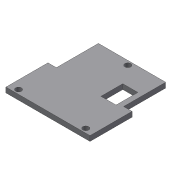
# Autodesk Inventor part: arm_0_bottom_case
Saved by Autodesk Inventor 2018 (Build 220112000, 112)
## iProperties
Created: 2017-12-04
Part Number: arm_0_bottom_case
Material: Generic
Document SubType Name: Modeling
Designer: Bardo91
Density: 1 g/cm^3
Appearance: Default
Mass: 6.66341 g
Surface Area: 51.4123 cm^2
Volume: 6.66341 cm^3
Author: Bardo91
Autodesk Inventor part; units mm, degrees
ref_plane "YZ Plane" through (0, 0, 0) normal (1, 0, 0) x (0, 1, 0)
ref_plane "XZ Plane" through (0, 0, 0) normal (0, 1, 0) x (-1, 0, 0)
ref_plane "XY Plane" through (0, 0, 0) normal (0, 0, 1) x (1, 0, 0)
sketch "Sketch1" plane through (0, 0, 0) normal (0, 0, 1) x (1, 0, 0)
  line L0 (0, 0) -> (50, 0)
  line L1 (50, 0) -> (50, 50)
  line L2 (50, 50) -> (0, 50)
  line L3 (0, 50) -> (0, 0)
  line L4 (25, 50) -> (25, 47.5)
  line L5 (0, 0) -> (5, 0)
  line L6 (5, 0) -> (5, 2.5)
  line L7 (50, 0) -> (45, 0)
  line L8 (45, 0) -> (45, 2.5)
  circle A0 centre (5, 2.5) radius 1.75
  circle A1 centre (45, 2.5) radius 1.75
  circle A2 centre (25, 47.5) radius 1.75
  line L9 (50, 50) -> (37, 50)
  line L10 (37, 50) -> (37, 30)
  line L11 (37, 30) -> (33, 30)
  line L12 (33, 30) -> (33, 23.5)
  line L13 (33, 23.5) -> (42, 23.5)
  line L14 (42, 23.5) -> (42, 36.5)
  line L15 (42, 36.5) -> (33, 36.5)
  line L16 (33, 36.5) -> (33, 30)
  dimension "d0" = 50
  dimension "d1" = 50
  dimension "d2" = 2.5
  dimension "d3" = 5
  dimension "d4" = 2.5
  dimension "d5" = 5
  dimension "d6" = 2.5
  dimension "d7" = 3.5
  dimension "d8" = 3.5
  dimension "d9" = 3.5
  dimension "d18" = 13
  dimension "d19" = 20
  dimension "d20" = 4
  dimension "d21" = 6.5
  dimension "d22" = 9
  dimension "d23" = 13
  dimension "d24" = 9
  constraints: 34 end point, 8 perpendicular, 4 point on line, 3 centre point, 3 coincident, 2 parallel, 1 horizontal, 1 midpoint, 1 vertical
  measures "d0" distance of L2.end L1.end
  measures "d1" distance of L1.end L0.end
  measures "d2" distance of L4.start L4.end
  measures "d3" distance of L0.start L5.end
  measures "d4" distance of L5.end L6.end
  measures "d5" distance of L0.end L7.end
  measures "d6" distance of L7.end L8.end
  measures "d7" diameter of A0
  measures "d8" diameter of A1
  measures "d9" diameter of A2
  measures "d18" distance of L1.end L9.end
  measures "d19" distance of L9.end L10.end
  measures "d20" distance of L10.end L11.end
  measures "d21" distance of L11.end L12.end
  measures "d22" distance of L12.end L13.end
  measures "d23" distance of L13.end L14.end
  measures "d24" distance of L14.end L15.end
extrude "Extrusion1" add sketch "Sketch1" along normal blind 3
sketch "Sketch2" plane through (0, 0, 3) normal (0, 0, 1) x (1, 0, 0)
  line L0 (50, 50) -> (0, 50) projected
  line L1 (0, 50) -> (5, 50)
  line L2 (5, 50) -> (5, 25)
  line L3 (5, 25) -> (0, 25)
  line L4 (0, 50) -> (0, 0) projected
  line L5 (0, 25) -> (0, 50)
  line L6 (0, 50) -> (0, 25)
  line L7 (50, 0) -> (50, 50) projected
  line L8 (50, 50) -> (50, 25)
  line L9 (50, 25) -> (45, 25)
  line L10 (45, 25) -> (45, 50)
  line L11 (45, 50) -> (50, 50)
  dimension "d12" = 5
  dimension "d13" = 25
  dimension "d14" = 25
  dimension "d15" = 5
  constraints: 18 end point, 4 perpendicular, 3 point on line, 2 collinear, 1 midpoint
  measures "d12" distance of L0.end L1.end
  measures "d13" distance of L1.end L2.end
  measures "d14" distance of L0.start L8.end
  measures "d15" distance of L8.end L9.end
extrude "Extrusion2" cut sketch "Sketch2" against normal through all
body "Solid1"
